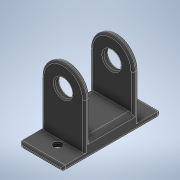
# Autodesk Inventor part: Bearing Block
Saved by Autodesk Inventor 2022 (Build 260153000, 153)
## iProperties
Created: 2021-12-04
Part Number: Bearing Block
Material: Generic
Document SubType Name: Modeling
Designer: LEGION SMIT
Density: 1 g/cm^3
Appearance: Generic
Author: LEGION SMIT
Autodesk Inventor part; units mm, degrees
ref_plane "YZ Plane" through (0, 0, 0) normal (1, 0, 0) x (0, 1, 0)
ref_plane "XZ Plane" through (0, 0, 0) normal (0, 1, 0) x (-1, 0, 0)
ref_plane "XY Plane" through (0, 0, 0) normal (0, 0, 1) x (1, 0, 0)
sketch "Sketch1" plane through (0, 0, 0) normal (1, 0, 0) x (0, 1, 0)
  line L0 (31.25, 10) -> (16.25, 10)
  line L1 (16.25, -10) -> (31.25, -10)
  line L2 (32.5, -12.5) -> (1.25, -12.5)
  line L3 (1.25, 12.5) -> (32.5, 12.5)
  line L4 (1.25, 22.5) -> (-1.25, 22.5)
  line L5 (1.25, -22.5) -> (-1.25, -22.5)
  line L6 (1.25, -22.5) -> (1.25, -12.5)
  line L7 (1.25, 12.5) -> (1.25, 22.5)
  line L8 (-1.25, 22.5) -> (-1.25, 10)
  line L9 (-1.25, -10) -> (-1.25, -22.5)
  line L10 (-1.25, -12.5) -> (-1.25, -10)
  line L11 (-1.25, 10) -> (-1.25, 12.5)
  line L12 (-1.25, 10) -> (-1.25, -10)
  line L13 (31.25, 10) -> (32.5, 10)
  line L14 (31.25, -10) -> (32.5, -10)
  line L15 (32.5, 12.5) -> (32.5, 10)
  line L16 (32.5, -10) -> (32.5, -12.5)
  line L17 (16.25, -10) -> (6.25, -10)
  line L18 (6.25, -10) -> (6.25, 10)
  line L19 (6.25, 10) -> (16.25, 10)
  dimension "d0" = 2.5
  dimension "d1" = 45
  dimension "d31" = 10
  constraints: 40 end point, 8 perpendicular, 7 parallel, 4 horizontal, 1 collinear
  measures "d0" distance of L4.end L4.start
  measures "d1" distance of L4.start L5.start
  measures "d31" distance of L1.start L17.end
extrude "Extrusion1" add sketch "Sketch1" along normal mid plane 20
fillet "Fillet1" radius 10 4 edges at (-10, 32.5, -11.25) (10, 32.5, -11.25) (10, 32.5, 11.25) (-10, 32.5, 11.25)
sketch "Sketch2" plane through (0, 22.5, -12.5) normal (0, 0, -1) x (-1, 0, 0)
  arc A0 (10, 0) -> (-10, 0) centre (0, 0) ccw projected
  circle A1 centre (0, 0) radius 4
  point P0 (0, -22.5)
  dimension "d10" = 8
  constraints: 1 centre point, 1 coincident
  measures "d10" diameter of A1
extrude "Extrusion2" cut sketch "Sketch2" against normal through all
fillet "Fillet2" radius 1 20 edges at (10, 11.8751, 12.5) (7.0711, 29.5711, 12.5) (0, 32.5, 12.5) (-7.0711, 29.5711, 12.5) (-10, 11.8751, 12.5) (10, 11.8751, -12.5) (7.0711, 29.5711, -12.5) (0, 32.5, -12.5) (-7.0711, 29.5711, -12.5) (-10, 11.8751, -12.5) (7.0711, 29.5711, -10) (-7.0711, 29.5711, -10) (0, 32.5, -10) (-10, 14.3751, -10) (10, 14.3751, -10) (0, 32.5, 10) (7.0711, 29.5711, 10) (-7.0711, 29.5711, 10) (-10, 14.3751, 10) (10, 14.3751, 10)
fillet "Fillet3" radius 1 10 edges at (0, 1.25, 22.5) (10, 0, 22.5) (-10, 0, 22.5) (0, -1.25, 22.5) (-10, 0, -22.5) (10, 0, -22.5) (0, 1.25, -22.5) (0, -1.25, -22.5) (10, -1.25, 0) (-10, -1.25, 0)
sketch "Sketch3" plane through (-9, -1.25, 21.5) normal (0, -1, 0) x (1, 0, 0)
  line L0 (9, -21.5) -> (9, -36.5)
  line L1 (9, -21.5) -> (9, -6.5)
  dimension "d16" = 15
  dimension "d19" = 15
  constraints: 4 end point, 2 vertical
  measures "d16" distance of L0.start L0.end
  measures "d19" distance of L0.start L1.end
hole "Hole1" at (0, -1.25, -15) at (0, -1.25, 15) direction (0, 1, 0) diameter 4 depth 6
thread "Thread1" size "M4x0.7" class "6H" standard "ANSI Metric M Profile" length 23.2
thread "Thread2" size "M4x0.7" class "6H" standard "ANSI Metric M Profile" length 23.2
fillet "Fillet4" radius 2 2 edges at (10, 6.25, 0) (-10, 6.25, 0)
fillet "Fillet5" radius 0.5 4 edges at (4, 22.5, 12.5) (4, 22.5, 10) (4, 22.5, -10) (4, 22.5, -12.5)
body "Solid1"
